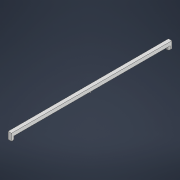
# Autodesk Inventor part: McCrea_otočka_walle
Saved by Autodesk Inventor 2022 (Build 260153000, 153)
## iProperties
Created: 2022-02-09
Part Number: McCrea_otočka_walle
Material: Generic
Document SubType Name: Modeling
Designer: MatusBarany
Density: 1 g/cm^3
Appearance: Default
Author: MatusBarany
Autodesk Inventor part; units mm, degrees
ref_plane "YZ Plane" through (0, 0, 0) normal (1, 0, 0) x (0, 1, 0)
ref_plane "XZ Plane" through (0, 0, 0) normal (0, 1, 0) x (-1, 0, 0)
ref_plane "XY Plane" through (0, 0, 0) normal (0, 0, 1) x (1, 0, 0)
sketch "Sketch1" plane through (0, 0, 0) normal (0, 1, 0) x (-1, 0, 0)
  line L0 (0, 225) -> (0, -225) construction
  line L1 (5, 225) -> (5, -225)
  line L2 (-5, -225) -> (-5, 225)
  arc A0 (5, 225) -> (-5, 225) centre (0, 225) ccw
  arc A1 (-5, -225) -> (5, -225) centre (0, -225) ccw
  circle A2 centre (0, 0) radius 2.5
  dimension "d0" = 450
  dimension "d1" = 10
  dimension "d2" = 5
  constraints: 8 end point, 4 point on circle, 4 tangent, 3 centre point, 1 coincident, 1 midpoint, 1 parallel, 1 vertical
  measures "d0" distance of L0.start L0.end
  measures "d1" distance between parallel lines of L1 L2
  measures "d2" diameter of A2
extrude "Extrusion1" add sketch "Sketch1" along normal blind 10 contours L1 A1 L2 A0 | A2
sketch "Sketch2" plane through (0, 0, 0) normal (0, -1, 0) x (1, 0, 0)
  circle A0 centre (0, 0) radius 2.5
  dimension "d5" = 5
  constraints: 1 centre point, 1 coincident
  measures "d5" diameter of A0
extrude "Extrusion2" add sketch "Sketch2" along normal blind 5
sketch "Sketch3" plane through (0, 10, 0) normal (0, 1, 0) x (1, 0, 0)
  line L0 (-5, 225) -> (-5, -225) projected
  arc A0 (-5, -225) -> (5, -225) centre (0, -225) ccw projected
  line L1 (5, -225) -> (5, 225) projected
  arc A1 (5, 225) -> (-5, 225) centre (0, 225) ccw projected
  circle A2 centre (0, -225) radius 5
  circle A3 centre (0, 225) radius 5
  line L2 (-5, -230) -> (5, -230)
  line L3 (5, -230) -> (5, -220)
  line L4 (5, -220) -> (-5, -220)
  line L5 (-5, -220) -> (-5, -230)
  line L6 (-5, 225) -> (-5, -225) projected
  line L7 (-5, 220) -> (5, 220)
  line L8 (5, 220) -> (5, 230)
  line L9 (5, 230) -> (-5, 230)
  line L10 (-5, 230) -> (-5, 220)
  point P0 (0, 0)
  point P1 (5, 225)
  point P2 (5, -225)
  point P3 (-5, -225)
  point P4 (0, 230)
  point P5 (5, 225)
  point P6 (-5, -225)
  point P7 (0, -230)
  point P8 (5, -225)
  dimension "d8" = 10
  dimension "d9" = 10
  constraints: 16 end point, 6 tangent, 4 parallel, 2 centre point, 2 coincident, 2 horizontal, 2 perpendicular, 2 point on line
  measures "d8" diameter of A2
  measures "d9" diameter of A3
extrude "Extrusion3" add sketch "Sketch3" against normal blind 20 contours L10 L9 A1 | A1 A3 | L9 L8 A1 | A2 A0 | A0 L2 L5 | A0 L3 L2
body "Solid1"
